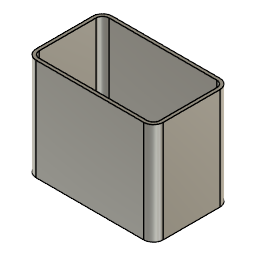
▢-125×75×3.2 (Autodesk Fusion 360 design; units mm, degrees)
Autodesk Fusion 360 part; units mm, degrees
sketch "スケッチ1" plane through (0, 0, 0) normal (0, 0, 1) x (1, 0, 0)
  line L0 (247.1191, -287.1642) -> (352.9191, -287.1642)
  line L1 (352.9191, -215.3642) -> (247.1191, -215.3642)
  line L2 (352.9191, -218.5642) -> (247.1191, -218.5642)
  line L3 (237.5191, -224.9642) -> (237.5191, -280.7642)
  line L4 (240.7191, -224.9642) -> (240.7191, -280.7642)
  arc A0 (240.7191, -280.7642) -> (247.1191, -287.1642) centre (247.1191, -280.7642) ccw
  arc A1 (247.1191, -215.3642) -> (237.5191, -224.9642) centre (247.1191, -224.9642) ccw
  arc A2 (247.1191, -218.5642) -> (240.7191, -224.9642) centre (247.1191, -224.9642) ccw
  line L5 (362.5191, -280.7642) -> (362.5191, -224.9642)
  line L6 (359.3191, -280.7642) -> (359.3191, -224.9642)
  arc A3 (352.9191, -287.1642) -> (359.3191, -280.7642) centre (352.9191, -280.7642) ccw
  arc A4 (362.5191, -224.9642) -> (352.9191, -215.3642) centre (352.9191, -224.9642) ccw
  arc A5 (359.3191, -224.9642) -> (352.9191, -218.5642) centre (352.9191, -224.9642) ccw
  line L7 (247.1191, -290.3642) -> (352.9191, -290.3642)
  arc A6 (237.5191, -280.7642) -> (247.1191, -290.3642) centre (247.1191, -280.7642) ccw
  arc A7 (352.9191, -290.3642) -> (362.5191, -280.7642) centre (352.9191, -280.7642) ccw
  point P0 (300.0191, -252.8642)
extrude "押し出し1" add sketch "スケッチ1" along normal blind 100
